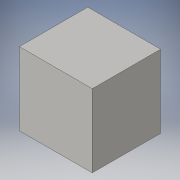
# Autodesk Inventor part: MC_DB1627
Saved by Autodesk Inventor 2016 (Build 200138000, 138)
## iProperties
Created: 2016-08-30
Part Number: MC_DB1627
Material: Generic
Document SubType Name: Modeling
Designer: jfixelle
Density: 1 g/cm^3
Appearance: Default
Author: jfixelle
Autodesk Inventor part; units mm, degrees
ref_plane "YZ Plane" through (0, 0, 0) normal (1, 0, 0) x (0, 1, 0)
ref_plane "XZ Plane" through (0, 0, 0) normal (0, 1, 0) x (-1, 0, 0)
ref_plane "XY Plane" through (0, 0, 0) normal (0, 0, 1) x (1, 0, 0)
sketch "Sketch1" plane through (0, 0, 0) normal (0, 1, 0) x (-1, 0, 0)
  line L0 (1.905, 2.03) -> (-2.155, 2.03)
  line L1 (-2.155, 2.03) -> (-2.155, -1.78)
  line L2 (-2.155, -1.78) -> (1.905, -1.78)
  line L3 (1.905, -1.78) -> (1.905, 2.03)
  point P0 (0, 0)
  dimension "d0" = 4.06
  dimension "d1" = 3.81
  dimension "d2" = 1.905
  dimension "d3" = 2.03
  constraints: 8 end point, 2 parallel, 1 horizontal, 1 perpendicular
  measures "d0" distance of L0.start L0.end
  measures "d1" distance of L2.end L0.start
  measures "d2" distance from line of point (0, 0) L3
  measures "d3" distance from line of point (0, 0) L0
extrude "Extrusion1" add sketch "Sketch1" along normal blind 4.06
body "Solid1"
